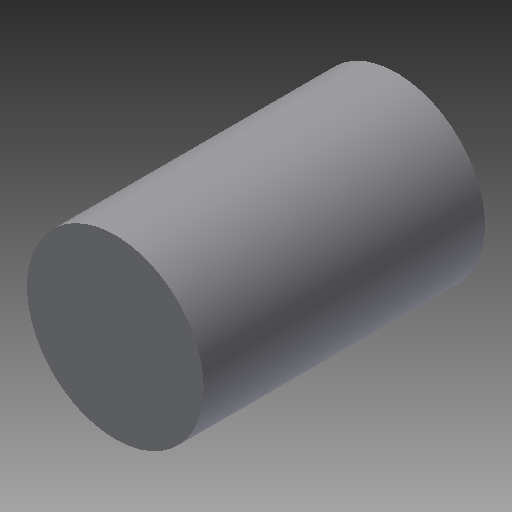
# Autodesk Inventor part: Pneumatics_VIAIR_00090_03
Saved by Autodesk Inventor 2017 (Build 210142000, 142)
## iProperties
Created: 2011-11-28
Part Number: Pneumatics_VIAIR_00090_03
Material: Generic
Document SubType Name: Modeling
Designer: Phillip
Density: 1 g/cm^3
Appearance: Default
Mass: 192.414 g
Surface Area: 188.727 cm^2
Volume: 192.414 cm^3
Author: Phillip
Autodesk Inventor part; units mm, degrees
ref_plane "YZ Plane" through (0, 0, 0) normal (1, 0, 0) x (0, 1, 0)
ref_plane "XZ Plane" through (0, 0, 0) normal (0, 1, 0) x (-1, 0, 0)
ref_plane "Work Plane1" through (-26.797, -37.3063, 85.979) normal (0, 0, -1) x (0, 1, 0)
sketch "Sketch1" plane through (0, 0, 0) normal (0, 0, 1) x (1, 0, 0)
  arc A0 (-23.9286, -16.5336) -> (-20.447, -28.194) centre (-20.447, -21.844) ccw projected
  line L0 (-20.447, -28.194) -> (20.447, -28.194) projected
  arc A1 (20.447, -28.194) -> (23.9286, -16.5336) centre (20.447, -21.844) ccw projected
  arc A2 (23.4121, -14.4336) -> (23.9286, -16.5336) centre (24.799, -15.206) ccw projected
  arc A3 (23.4121, -14.4336) -> (26.797, -1.397) centre (0, -1.397) ccw projected
  line L1 (26.797, -1.397) -> (26.797, 19.05) projected
  arc A4 (26.797, 19.05) -> (20.447, 25.4) centre (20.447, 19.05) ccw projected
  line L2 (20.447, 25.4) -> (-20.447, 25.4) projected
  arc A5 (-20.447, 25.4) -> (-26.797, 19.05) centre (-20.447, 19.05) ccw projected
  line L3 (-26.797, 19.05) -> (-26.797, -1.397) projected
  arc A6 (-26.797, -1.397) -> (-23.4121, -14.4336) centre (0, -1.397) ccw projected
  arc A7 (-23.9286, -16.5336) -> (-23.4121, -14.4336) centre (-24.799, -15.206) ccw projected
  circle A8 centre (0, -1.397) radius 26.797
  point P0 (0, 0)
  dimension "d0" = 53.594
  constraints: 1 centre point, 1 coincident
  measures "d0" diameter of A8
extrude "Extrusion1" add sketch "Sketch1" along normal blind 85.2932 contours A6 A8 A3
body "Solid1"
